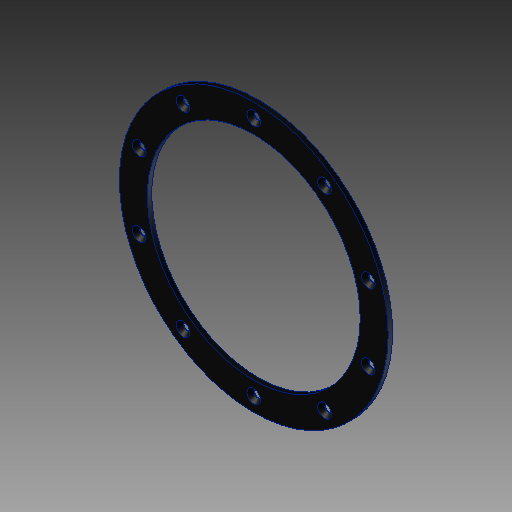
# Autodesk Inventor part: 1134_RU O Ring Cap_V1
Saved by Autodesk Inventor 2020 (Build 240168000, 168)
## iProperties
Created: 2019-03-29
Part Number: 1134_RU O Ring Cap_V1
Material: Aluminum 6061
Document SubType Name: Modeling
Designer: e22ma
Density: 2.7 g/cm^3
Appearance: Aluminum - Flat
Mass: 89.3413 g
Surface Area: 250.708 cm^2
Volume: 33.0894 cm^3
Author: e22ma
Autodesk Inventor part; units mm, degrees
ref_plane "YZ Plane" through (0, 0, 0) normal (1, 0, 0) x (0, 1, 0)
ref_plane "XZ Plane" through (0, 0, 0) normal (0, 1, 0) x (-1, 0, 0)
ref_plane "XY Plane" through (0, 0, 0) normal (0, 0, 1) x (1, 0, 0)
sketch "Sketch1" plane through (0, 0, 0) normal (0, 0, 1) x (1, 0, 0)
  circle A0 centre (0, 0) radius 76.2
  circle A1 centre (0, 0) radius 96.2
  dimension "d0" = 152.4
  dimension "d1" = 20
  constraints: 2 centre point, 1 coincident
  measures "d0" diameter of A0
  measures "d1" radial gap between concentric circles of A0 A1
extrude "Extrusion1" add sketch "Sketch1" along normal blind 3.175
sketch "Sketch2" plane through (0, 0, 3.175) normal (0, 0, 1) x (1, 0, 0)
  circle A0 centre (0, 0) radius 76.2 projected
  circle A1 centre (0, 0) radius 96.2 projected
  circle A2 centre (0, 0) radius 76.2 projected
  line L0 (0, 76.2) -> (0, 96.2)
  point P0 (0, 86.2)
  point P1 (0, 86.2)
  constraints: 3 vertical alignment, 2 end point, 1 coincident, 1 midpoint, 1 vertical, 2 other
hole "Hole1" at (0, 86.2, 3.175) direction (0, 0, -1) diameter 4.978 depth 8 tip angle 118 countersink diameter 9.779 countersink angle 82 clearance for "Flat Head Machine Screw (82)" size "#10" standard "Ansi Unified Screw Threads"
pattern_circular "Circular Pattern1" count 10 over 360 about axis through (0, 0, 0) along (0, 0, 1) of "Hole1"
body "Solid1"
